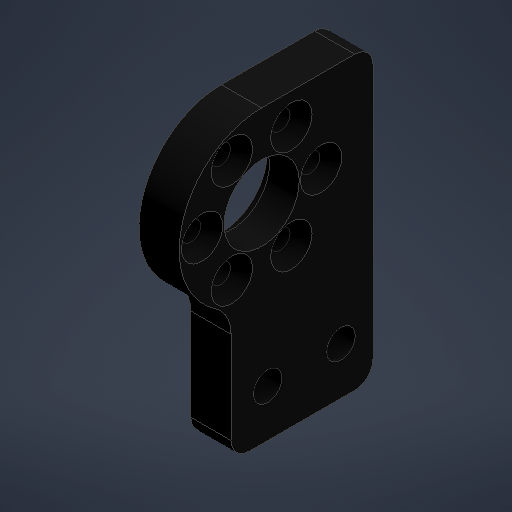
# Autodesk Inventor part: Motorhalterung
Saved by Autodesk Inventor 2025.2 (Build 292293000, 293)
## iProperties
Created: 2024-11-27
Part Number: Motorhalterung
Material: Generisch
Document SubType Name: Modeling
Designer: Fabian
Density: 1 g/cm^3
Appearance: Vorgabe
Author: Fabian
Autodesk Inventor part; units mm, degrees
ref_plane "YZ Plane" through (0, 0, 0) normal (1, 0, 0) x (0, 1, 0)
sketch "Skizze1" plane through (0, 0, 0) normal (1, 0, 0) x (0, 1, 0)
  circle A0 centre (-14.5, 4) radius 1.2295
  circle A1 centre (-14.5, 4) radius 1.6
  circle A2 centre (-14.5, -4) radius 1.2295
  circle A3 centre (-14.5, -4) radius 1.6
  circle A4 centre (0, 0) radius 8
  circle A5 centre (0, 0) radius 5
  line L0 (0, 8) -> (-18.5, 8)
  line L1 (0, -8) -> (-18.5, -8)
  line L2 (-18.5, -8) -> (-18.5, 8)
  circle A6 centre (0, 0) radius 5.2
  circle A7 centre (0, 0) radius 9
  circle A8 centre (0, 0) radius 4.1
  line L3 (0, 8) -> (-17.478, 8)
  line L4 (-17.478, 8) -> (-17.478, -8)
  line L5 (-14.5, 4) -> (-17.478, 4)
  line L6 (-14.5, -4) -> (-17.478, -4)
  circle A9 centre (-17.478, 4) radius 1.55
  circle A10 centre (-17.478, -4) radius 1.55
  line L7 (-17.478, 4) -> (-21.478, 4)
  line L8 (-21.478, 4) -> (-21.478, 8)
  line L9 (-21.478, 8) -> (-18.5, 8)
  line L10 (-18.5, 8) -> (-21.478, 8)
  line L11 (-21.478, 8) -> (-21.478, -8)
  line L12 (-21.478, -8) -> (-18.5, -8)
  line L13 (-18.5, -8) -> (-18.5, 8)
  point P0 (0, 6.5)
  point P1 (-5.6292, 3.25)
  point P2 (-5.6292, -3.25)
  point P3 (0, -6.5)
  point P4 (5.6292, -3.25)
  point P5 (5.6292, 3.25)
  point P6 (-4.1231, 8)
  point P7 (-4.1231, -8)
  dimension "d2" = 3.2
  dimension "d3" = 3.2
  dimension "d4" = 16
  dimension "d5" = 10
  dimension "d6" = 360
  dimension "d7" = 0.2
  dimension "d17" = 1
  dimension "d20" = 8.2
  dimension "d73" = 17.478
  dimension "d74" = 3.1
  dimension "d75" = 3.1
  dimension "d76" = 4
  constraints: 28 end point, 11 centre point, 8 coincident, 6 perpendicular, 4 point on line, 2 horizontal, 2 parallel, 2 point on circle, 7 other
  measures "d2" diameter of A1
  measures "d3" diameter of A3
  measures "d4" diameter of A4
  measures "d5" diameter of A5
  measures "d7" radial gap between concentric circles of A5 A6
  measures "d17" radial gap between concentric circles of A4 A7
  measures "d20" diameter of A8
  measures "d73" distance of L0.start L3.end
  measures "d74" diameter of A9
  measures "d75" diameter of A10
  measures "d76" distance of L7.start L7.end
extrude "Extrusion1" add sketch "Skizze1" against normal blind 3 contours A0 | A1 A9 | A1 A9 L4 L0 A7 L1 A10 A3 | A9 L2 L0 L4 | L4 A10 L2 A9 | A9 L7 L8 L9 L2 | L2 A10 L12 L11 L7 A9 | A7 L1 A4 L0 | L0 A4 L1 A7 | A3 A10 | A4 | L4 L1 L2 A10 | A2 | A5 | A6
fillet "Rundung1" radius 4 2 edges at (-1.5, -4.1231, 8) (-1.5, -4.1231, -8)
fillet "Rundung2" radius 2 2 edges at (-1.5, -21.478, 8) (-1.5, -21.478, -8)
ref_plane "Arbeitsebene1" through (-0.25, 0, 0) normal (1, 0, 0) x (0, 0, -1)
sketch "Skizze6" plane through (0, 0, 0) normal (1, 0, 0) x (0, 0, -1)
  circle A0 centre (-4, -17.478) radius 1.55 projected
  line L0 (-4, -17.478) -> (-4, -9.678)
  line L1 (-4, -9.678) -> (-14.914, -9.678)
  circle A1 centre (-14.914, -9.678) radius 9
  point P0 (0, 0)
  dimension "d79" = 7.8
  dimension "d80" = 10.914
  dimension "d81" = 18
  constraints: 4 end point, 1 centre point, 1 coincident, 1 perpendicular, 1 vertical
  measures "d79" distance of L0.start L0.end
  measures "d80" distance of L0.end L1.end
  measures "d81" diameter of A1
extrude "Extrusion4" cut sketch "Skizze6" against normal blind 3 contours A1
fillet "Rundung3" radius 2 2 edges at (-1.5, -3.6438, 8.2365) (-1.5, -15.4396, 8)
sketch "Skizze8" plane through (-3, 0, 0) normal (-1, 0, 0) x (0, 0, 1)
  circle A0 centre (0, 0) radius 8
  circle A1 centre (-0.6675, -17.6407) radius 2.1
  circle A2 centre (-0.6675, -17.6407) radius 2.1
  circle A3 centre (-8.6675, -17.6407) radius 2.1
  circle A4 centre (-8.6675, -17.6407) radius 2.1
  line L0 (-0.6675, -17.6407) -> (-8.6675, -17.6407)
  line L1 (0, -8) -> (-4.6675, -8)
  line L2 (-4.6675, 8) -> (0, 8)
  arc A5 (0, -8) -> (0, 8) centre (0, 0) ccw
  arc A6 (-4.6675, 8) -> (-4.6675, -8) centre (-4.6675, 0) ccw
  line L3 (1.3325, -22.7814) -> (-10.6675, -22.7814)
  line L4 (-12.6675, -20.7814) -> (-12.6675, 0)
  line L5 (-4.6675, 8) -> (0, 8)
  line L6 (3.3325, 7.2729) -> (3.3325, -20.7814)
  arc A7 (1.3325, -22.7814) -> (3.3325, -20.7814) centre (1.3325, -20.7814) ccw
  arc A8 (-12.6675, -20.7814) -> (-10.6675, -22.7814) centre (-10.6675, -20.7814) ccw
  circle A9 centre (0, 0) radius 9
  line L7 (0, 0) -> (-4.6675, 0) construction
  line L8 (0, -9) -> (-4.6675, -9)
  line L9 (-4.6675, 9) -> (0, 9)
  arc A10 (0, -9) -> (0, 9) centre (0, 0) ccw
  arc A11 (-4.6675, 9) -> (-4.6675, -9) centre (-4.6675, 0) ccw
  line L10 (-12.6675, 0) -> (-12.6675, 4.1231)
  line L11 (13.9828, -24.3556) -> (-18.0791, -24.3556)
  line L12 (-18.0791, -24.3556) -> (-18.0791, 10.5895)
  line L13 (-18.0791, 10.5895) -> (13.9828, 10.5895)
  line L14 (13.9828, 10.5895) -> (13.9828, -24.3556)
  arc A12 (8.0333, -3.8766) -> (7.6207, -14.9513) centre (14.914, -9.678) ccw projected
  circle A13 centre (14.914, -9.678) radius 9
  arc A14 (8.0333, -3.8766) -> (8.3626, -3.3267) centre (6.5042, -2.5875) ccw projected
  arc A15 (8.0333, -3.8766) -> (8.3626, -3.3267) centre (6.5042, -2.5875) ccw
  line L15 (-13.6675, 0) -> (-13.6675, -22.7814)
  line L16 (-13.6675, -22.7814) -> (-10.6675, -22.7814)
  point P0 (-2.3338, 0)
  point P1 (-12.6675, -4.1231)
  point P2 (3.3325, -8.3603)
  point P3 (8.2224, -3.6594)
  point P4 (8.0333, -3.8766)
  point P5 (6.6916, -6.0186)
  point P6 (8.0333, -3.8766)
  dimension "d88" = 16
  dimension "d90" = 2
  constraints: 36 end point, 18 point on circle, 14 tangent, 13 centre point, 6 parallel, 5 coincident, 4 horizontal, 3 perpendicular, 2 equal radius, 2 vertical, 1 midpoint, 2 other
  measures "d88" diameter of A0
  measures "d90" radius of A7
extrude "Extrusion5" cut sketch "Skizze8" against normal blind 3 contours A9 A12 A13 L14 L11 L12 L13 L9 A11 L15 L16 L3 A7 L6 | A9 A13 L14 A12 | L16 L15 A11 L4 A8
extrude "Extrusion6" add sketch "Skizze8" against normal blind 3 contours A12 A13 A9 | A13 A14 A9
extrude "Extrusion7" add sketch "Skizze8" against normal up to surface (3 mm away) contours L6 A7 L3 A8 L4 A11 L8 A9 | A9 L1 A6 L2 | L2 A6 L10 A11 L9 A9 | A9 L8 A11 L4 A6 L1 | L4 A11 L10 | L16 L15 A11 L4 A8 | A1 | A3
extrude "Extrusion8" cut sketch "Skizze8" against normal up to surface (3 mm away) contours A1 | A3
fillet "Rundung4" radius 4 1 edges at (-1.5, -8.3603, 3.3325)
sketch "Skizze10" plane through (0, 0, 0) normal (1, 0, 0) x (0, 0, -1)
  circle A0 centre (0.6675, -17.6407) radius 2.1 projected
  circle A1 centre (0.6675, -17.6407) radius 1.55
  circle A2 centre (8.6675, -17.6407) radius 2.1 projected
  circle A3 centre (8.6675, -17.6407) radius 1.55
  circle A4 centre (0.6675, -17.6407) radius 2.1
  circle A5 centre (8.6675, -17.6407) radius 2.1
  point P0 (0, 0)
  dimension "d106" = 3.1
  dimension "d107" = 3.1
  constraints: 4 centre point, 4 coincident, 2 concentric
  measures "d106" diameter of A1
  measures "d107" diameter of A3
extrude "Extrusion10" add sketch "Skizze10" against normal up to surface (3 mm away)
sketch "Skizze11" plane through (-3, 0, 0) normal (-1, 0, 0) x (0, 0, 1)
  circle A0 centre (0, 0) radius 5
  circle A1 centre (-8.6675, -17.6407) radius 1.55 projected
  circle A2 centre (-0.6675, -17.6407) radius 1.55 projected
  line L0 (-4.6675, 9) -> (0, 9) projected
  arc A3 (5.0763, -7.4317) -> (0, 9) centre (0, 0) ccw projected
  arc A4 (5.0763, -7.4317) -> (3.3325, -10.7347) centre (7.3325, -10.7347) ccw projected
  line L1 (3.3325, -10.7347) -> (3.3325, -20.7814) projected
  arc A5 (1.3325, -22.7814) -> (3.3325, -20.7814) centre (1.3325, -20.7814) ccw projected
  circle A6 centre (0, 0) radius 4.1 projected
  line L2 (1.3325, -22.7814) -> (-13.6675, -22.7814) projected
  line L3 (-13.6675, -22.7814) -> (-13.6675, 0) projected
  arc A7 (-4.6675, 9) -> (-13.6675, 0) centre (-4.6675, 0) ccw projected
  point P0 (-8.0425, 8.3432)
  point P1 (-10.6675, -22.7814)
  point P2 (-12.6675, 4.1231)
  dimension "d110" = 10
  constraints: 1 centre point, 1 coincident
  measures "d110" diameter of A0
extrude "Extrusion11" add sketch "Skizze11" along normal blind 1.4 contours A0 | L0 A3 A4 L1 A5 L2 L3 A7
sketch "Skizze12" plane through (-4.4, 0, 0) normal (-1, 0, 0) x (0, 0, 1)
  circle A0 centre (0, 0) radius 5
  dimension "d115" = 10
  constraints: 1 centre point, 1 coincident
  measures "d115" diameter of A0
extrude "Extrusion13" cut sketch "Skizze12" against normal blind 1.15
ref_plane "Arbeitsebene2" through (-1.4, 0, 0) normal (-1, 0, 0) x (0, 0, 1)
sketch "Skizze16" plane through (0, 0, 0) normal (1, 0, 0) x (0, 0, -1)
  circle A0 centre (-4, -14.5) radius 1.2295
  circle A1 centre (-4, -14.5) radius 1.5
  circle A2 centre (4, -14.5) radius 1.2295
  circle A3 centre (4, -14.5) radius 1.5
  circle A4 centre (0, 0) radius 8
  circle A5 centre (0, 0) radius 5
  line L0 (-8, 0) -> (-8, -18.5)
  line L1 (8, 0) -> (8, -18.5)
  line L2 (8, -18.5) -> (-8, -18.5)
  circle A6 centre (0, 0) radius 5.2
  circle A7 centre (0, 0) radius 9
  circle A8 centre (0, 0) radius 4.1
  point P0 (0, 0)
  point P1 (0, 0)
  point P2 (0, 0)
  point P3 (0, 0)
  point P4 (-6.5, 0)
  point P5 (-3.25, -5.6292)
  point P6 (3.25, -5.6292)
  point P7 (6.5, 0)
  point P8 (3.25, 5.6292)
  point P9 (-3.25, 5.6292)
  point P10 (-59.3826, 46.4511)
  point P11 (-59.3826, 30.4511)
  dimension "d155" = 3
  dimension "d156" = 3
  dimension "d157" = 16
  dimension "d158" = 10
  dimension "d159" = 360
  dimension "d160" = 0.2
  dimension "d161" = 1
  dimension "d162" = 8.2
  constraints: 9 centre point, 6 coincident, 6 end point, 2 point on circle, 7 other
  measures "d155" diameter of A1
  measures "d156" diameter of A3
  measures "d157" diameter of A4
  measures "d158" diameter of A5
  measures "d160" radial gap between concentric circles of A5 A6
  measures "d161" radial gap between concentric circles of A4 A7
  measures "d162" diameter of A8
hole "Bohrung7" at (0, 0, 6.5) at (0, -5.6292, 3.25) at (0, -5.6292, -3.25) at (0, 0, -6.5) at (0, 5.6292, -3.25) at (0, 5.6292, 3.25) direction (-1, 0, 0) diameter 2.1 end through all countersink diameter 4.5 countersink angle 90
sketch "Skizze17" plane through (0, 0, 0) normal (1, 0, 0) x (0, 0, -1)
  arc A0 (13.6675, 0) -> (4.6675, 9) centre (4.6675, 0) ccw projected
  line L0 (4.6675, 9) -> (13.6675, 9)
  line L1 (13.6675, 9) -> (13.6675, -22.7814)
  line L2 (13.6675, -22.7814) -> (-1.3325, -22.7814) projected
  line L3 (13.6675, -22.7814) -> (12.1675, -22.7814)
  line L4 (12.1675, -22.7814) -> (12.1675, 9)
  circle A1 centre (-3.25, 5.6292) radius 2.25 projected
  circle A2 centre (3.25, 5.6292) radius 2.25 projected
  circle A3 centre (6.5, 0) radius 2.25 projected
  circle A4 centre (3.25, -5.6292) radius 2.25 projected
  circle A5 centre (-3.25, -5.6292) radius 2.25 projected
  circle A6 centre (-6.5, 0) radius 2.25 projected
  circle A7 centre (8.6675, -17.6407) radius 1.55 projected
  circle A8 centre (0.6675, -17.6407) radius 1.55 projected
  line L5 (0, 9) -> (4.6675, 9) projected
  arc A9 (13.6675, 0) -> (4.6675, 9) centre (4.6675, 0) ccw projected
  line L6 (13.6675, 0) -> (13.6675, -22.7814) projected
  line L7 (13.6675, -22.7814) -> (-1.3325, -22.7814) projected
  arc A10 (-3.3325, -20.7814) -> (-1.3325, -22.7814) centre (-1.3325, -20.7814) ccw projected
  line L8 (-3.3325, -20.7814) -> (-3.3325, -10.7347) projected
  arc A11 (-3.3325, -10.7347) -> (-5.0763, -7.4317) centre (-7.3325, -10.7347) ccw projected
  arc A12 (0, 9) -> (-5.0763, -7.4317) centre (0, 0) ccw projected
  circle A13 centre (0, 0) radius 4.1 projected
  point P0 (12.1675, 4.9749)
  dimension "d174" = 1.5
  constraints: 8 end point, 2 perpendicular, 2 point on line, 1 horizontal, 1 tangent
  measures "d174" distance of L1.end L3.end
extrude "Extrusion14" cut sketch "Skizze17" against normal through all contours L1 L2 L4 A0 | A0 L4 L0 L1
extrude "Extrusion15" add sketch "Skizze17" against normal up to surface (4.4 mm away) contours A0 L0 L4
fillet "Rundung7" radius 2 2 edges at (-2.2, 9, -12.1675) (-2.2, -22.7814, -12.1675)
